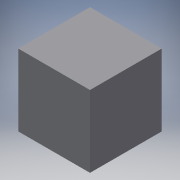
# Autodesk Inventor part: Glyph
Saved by Autodesk Inventor 2017 (Build 210142000, 142)
## iProperties
Created: 2017-09-30
Part Number: Glyph
Material: Generic
Document SubType Name: Modeling
Designer: Kenneth
Density: 1 g/cm^3
Appearance: Default
Author: Kenneth
Autodesk Inventor part; units mm, degrees
ref_plane "YZ Plane" through (0, 0, 0) normal (1, 0, 0) x (0, 1, 0)
ref_plane "XZ Plane" through (0, 0, 0) normal (0, 1, 0) x (-1, 0, 0)
ref_plane "XY Plane" through (0, 0, 0) normal (0, 0, 1) x (1, 0, 0)
sketch "Sketch1" plane through (0, 0, 0) normal (0, 1, 0) x (-1, 0, 0)
  line L0 (-76.2, 76.2) -> (76.2, 76.2)
  line L1 (76.2, 76.2) -> (76.2, -76.2)
  line L2 (76.2, -76.2) -> (-76.2, -76.2)
  line L3 (-76.2, -76.2) -> (-76.2, 76.2)
  line L4 (-76.2, 76.2) -> (76.2, -76.2) construction
  line L5 (76.2, 76.2) -> (-76.2, -76.2) construction
  point P0 (0, 0)
  dimension "d0" = 152.4
  dimension "d1" = 152.4
  constraints: 12 end point, 2 midpoint, 2 parallel, 1 horizontal, 1 perpendicular
  measures "d0" distance of L0.end L1.end
  measures "d1" distance of L1.end L2.end
extrude "Extrusion1" add sketch "Sketch1" along normal blind 152.4
body "Solid1"
